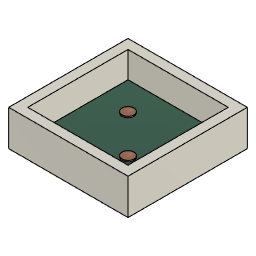
watch v61 (Autodesk Fusion 360 design; units mm, degrees)
Autodesk Fusion 360 part; units mm, degrees
sketch "Sketch2" plane through (0, 0, 0) normal (0, 0, 1) x (1, 0, 0)
  line L0 (-25, 25) -> (25, 25)
  line L1 (25, 25) -> (25, -25)
  line L2 (25, -25) -> (-25, -25)
  line L3 (-25, -25) -> (-25, 25)
  constraint horizontal L0
  constraint vertical L1
  constraint horizontal L2
  constraint vertical L3
extrude "Extrude1" add sketch "Sketch2" along normal blind 15 makes body 1 in component "Component"
shell "Shell1" thickness 4 removed faces 1 at (-8.3333, 8.3333, 15) on bodies 1 in component "Component"
sketch "Sketch3" plane through (0, 0, 4) normal (0, 0, 1) x (-1, 0, 0)
  line L0 (21, 21) -> (-21, 21)
  line L1 (-21, 21) -> (-21, -21)
  line L2 (-21, -21) -> (21, -21)
  line L3 (21, -21) -> (21, 21)
  line L4 (20, -20) -> (-20, -20)
  line L5 (-20, -20) -> (-20, 20)
  line L6 (-20, 20) -> (20, 20)
  line L7 (20, 20) -> (20, -20)
  constraint horizontal L4
  constraint vertical L5
  constraint horizontal L6
  constraint vertical L7
extrude "Extrude1'" add sketch "Sketch3" along normal blind 1 separate body contours L4 L5 L6 L7 makes body 2 in component "Component'"
sketch "Sketch1" plane through (0, 0, 5) normal (0, 0, 1) x (-1, 0, 0) in component "Component'"
  line L0 (20, 20) -> (-20, 20)
  line L1 (-20, 20) -> (-20, -20)
  line L2 (-20, -20) -> (20, -20)
  line L3 (20, -20) -> (20, 20)
  circle A0 centre (8, -8) radius 2.5
  circle A1 centre (-8, 8) radius 2.5
  dimension "d6" = 5
  dimension "d7" = 5
  measures "d6" diameter of A0
  measures "d7" diameter of A1
extrude "Extrude2" add sketch "Sketch1" along normal blind 0.5 separate body contours A0 | A1 makes body 3 at (-7.8146, 7.261, 5) makes body 4 at (7.8513, -8.6515, 5) in component "Component'"
component "Component" placed x (1, 0, 0) y (0, 1, 0) z (0, 0, 1) at (0, 0, 0)
component "Component'" placed x (1, 0, 0) y (0, 1, 0) z (0, 0, 1) at (0, 0, 0)
named bodies: "shell", "silicon", "source1", "source2"
